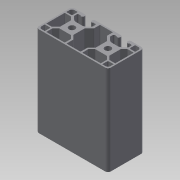
# Autodesk Inventor part: 40-4082-LITE
Saved by Autodesk Inventor 2013 (Build 170138000, 138)
## iProperties
Created: 2014-04-23
Part Number: 40-4082-LITE
Material: Generic
Document SubType Name: Modeling
Designer: Ross Bowman
Density: 1 g/cm^3
Engineer: Ross Bowman
Catalog Web Link: 8020.net
Vendor: 80/20 Inc.
Company: 80/20 Inc.
Author: Ross Bowman
Keywords: 80/20 , 8020 , T-Slot , Extrusion
Material: 6105-T5 Aluminum
Autodesk Inventor part; units mm, degrees
ref_plane "YZ Plane" through (0, 0, 0) normal (1, 0, 0) x (0, 1, 0)
ref_plane "XZ Plane" through (0, 0, 0) normal (0, 1, 0) x (-1, 0, 0)
ref_plane "XY Plane" through (0, 0, 0) normal (0, 0, 1) x (1, 0, 0)
sketch "Sketch1" plane through (0, 0, 0) normal (0, 0, 1) x (1, 0, 0)
  circle A0 centre (-20, 0) radius 3.3778
  circle A1 centre (20, 0) radius 3.3778
  arc A2 (31.462, -10.0253) -> (32.0906, -10.2857) centre (32.0906, -9.3967) ccw
  line L0 (27.9429, -6.5063) -> (31.462, -10.0253)
  arc A3 (27.6825, -5.8776) -> (27.9429, -6.5063) centre (28.5715, -5.8776) ccw
  line L1 (27.6825, 6.0573) -> (27.6825, -5.8776)
  arc A4 (27.9429, 6.6858) -> (27.6825, 6.0573) centre (28.5714, 6.0573) ccw
  line L2 (31.2824, 10.0254) -> (27.9429, 6.6858)
  arc A5 (31.911, 10.2857) -> (31.2824, 10.0254) centre (31.911, 9.3968) ccw
  line L3 (37.975, 10.2857) -> (31.911, 10.2857)
  line L4 (32.0906, -10.2857) -> (37.975, -10.2857)
  arc A6 (30.2857, -11.911) -> (30.0253, -11.2824) centre (29.3967, -11.911) ccw
  line L5 (30.2857, -17.975) -> (30.2857, -11.911)
  line L6 (9.7143, -11.911) -> (9.7143, -17.975)
  arc A7 (9.9746, -11.2824) -> (9.7143, -11.911) centre (10.6032, -11.911) ccw
  line L7 (13.3142, -7.9429) -> (9.9746, -11.2824)
  arc A8 (13.9427, -7.6825) -> (13.3142, -7.9429) centre (13.9427, -8.5714) ccw
  line L8 (26.0572, -7.6825) -> (13.9427, -7.6825)
  arc A9 (26.6858, -7.9429) -> (26.0572, -7.6825) centre (26.0572, -8.5715) ccw
  line L9 (30.0253, -11.2824) -> (26.6858, -7.9429)
  arc A10 (-26.0573, -7.6825) -> (-26.6858, -7.9429) centre (-26.0573, -8.5714) ccw
  line L10 (-13.9427, -7.6825) -> (-26.0573, -7.6825)
  arc A11 (-13.3142, -7.9429) -> (-13.9427, -7.6825) centre (-13.9427, -8.5714) ccw
  line L11 (-9.9746, -11.2824) -> (-13.3142, -7.9429)
  arc A12 (-9.7143, -11.911) -> (-9.9746, -11.2824) centre (-10.6032, -11.911) ccw
  line L12 (-9.7143, -17.975) -> (-9.7143, -11.911)
  line L13 (-30.2857, -11.911) -> (-30.2857, -17.975)
  arc A13 (-30.0254, -11.2824) -> (-30.2857, -11.911) centre (-29.3968, -11.911) ccw
  line L14 (-26.6858, -7.9429) -> (-30.0254, -11.2824)
  line L15 (-33.2063, -11.9365) -> (-37.975, -11.9365)
  arc A14 (-31.9365, -13.2063) -> (-33.2063, -11.9365) centre (-33.2063, -13.2063) ccw
  line L16 (-31.9365, -17.975) -> (-31.9365, -13.2063)
  line L17 (-31.9365, 13.2063) -> (-31.9365, 17.9355)
  arc A15 (-33.2063, 11.9365) -> (-31.9365, 13.2063) centre (-33.2063, 13.2063) ccw
  line L18 (-37.975, 11.9365) -> (-33.2063, 11.9365)
  arc A16 (-31.2824, 10.0254) -> (-31.911, 10.2857) centre (-31.911, 9.3968) ccw
  line L19 (-27.9429, 6.6858) -> (-31.2824, 10.0254)
  arc A17 (-27.6825, 6.0573) -> (-27.9429, 6.6858) centre (-28.5714, 6.0573) ccw
  line L20 (-27.6825, -5.5185) -> (-27.6825, 6.0573)
  arc A18 (-27.9429, -6.1471) -> (-27.6825, -5.5185) centre (-28.5714, -5.5185) ccw
  line L21 (-31.8212, -10.0254) -> (-27.9429, -6.1471)
  arc A19 (-32.4497, -10.2857) -> (-31.8212, -10.0254) centre (-32.4497, -9.3968) ccw
  line L22 (-37.975, -10.2857) -> (-32.4497, -10.2857)
  line L23 (-31.911, 10.2857) -> (-37.975, 10.2857)
  arc A20 (7.1746, 11.9365) -> (7.435, 11.308) centre (8.0635, 11.9365) ccw
  line L24 (12.0571, 6.6858) -> (7.435, 11.308)
  arc A21 (12.3175, 6.0573) -> (12.0571, 6.6858) centre (11.4286, 6.0573) ccw
  line L25 (12.3175, -5.8777) -> (12.3175, 6.0573)
  arc A22 (12.0571, -6.5062) -> (12.3175, -5.8777) centre (11.4286, -5.8777) ccw
  line L26 (8.0699, -10.4935) -> (12.0571, -6.5062)
  arc A23 (8.0699, -10.4935) -> (7.8095, -11.122) centre (8.6984, -11.122) ccw
  line L27 (7.8095, -17.975) -> (7.8095, -11.122)
  line L28 (-7.8095, -11.122) -> (-7.8095, -17.975)
  arc A24 (-7.8095, -11.122) -> (-8.0699, -10.4935) centre (-8.6984, -11.122) ccw
  line L29 (-12.0571, -6.5062) -> (-8.0699, -10.4935)
  arc A25 (-12.3175, -5.8777) -> (-12.0571, -6.5062) centre (-11.4286, -5.8777) ccw
  line L30 (-12.3175, 6.0573) -> (-12.3175, -5.8777)
  arc A26 (-12.0571, 6.6858) -> (-12.3175, 6.0573) centre (-11.4286, 6.0573) ccw
  line L31 (-7.435, 11.308) -> (-12.0571, 6.6858)
  arc A27 (-7.435, 11.308) -> (-7.1746, 11.9365) centre (-8.0635, 11.9365) ccw
  line L32 (-7.1746, 17.9355) -> (-7.1746, 11.9365)
  line L33 (35.56, 18.3105) -> (32.3115, 18.3105)
  line L34 (7.1746, 11.9365) -> (7.1746, 17.9355)
  line L35 (31.9365, -13.2063) -> (31.9365, -17.975)
  arc A28 (33.2063, -11.9365) -> (31.9365, -13.2063) centre (33.2063, -13.2063) ccw
  line L36 (37.975, -11.9365) -> (33.2063, -11.9365)
  line L37 (33.2063, 11.9365) -> (37.975, 11.9365)
  arc A29 (31.9365, 13.2063) -> (33.2063, 11.9365) centre (33.2063, 13.2063) ccw
  line L38 (31.9365, 17.9355) -> (31.9365, 13.2063)
  arc A30 (36.8254, -20) -> (40, -16.8254) centre (36.8254, -16.8254) ccw
  line L39 (40, -16.8254) -> (40, 16.8254)
  arc A31 (40, 16.8254) -> (36.8254, 20) centre (36.8254, 16.8254) ccw
  line L40 (36.8254, 20) -> (25.6381, 20)
  arc A32 (25.6381, 20) -> (24.0635, 18.4254) centre (25.6381, 18.4254) ccw
  line L41 (24.0635, 18.4254) -> (24.0635, 17.5111)
  arc A33 (24.0635, 17.5111) -> (25.6381, 15.9365) centre (25.6381, 17.5111) ccw
  line L42 (25.6381, 15.9365) -> (26.3446, 15.9365)
  arc A34 (26.3446, 15.9365) -> (26.7243, 16.3032) centre (26.3446, 16.3165) ccw
  line L43 (26.7243, 16.3032) -> (26.7253, 16.3317)
  arc A35 (27.105, 16.6984) -> (26.7253, 16.3317) centre (27.105, 16.3185) ccw
  line L44 (27.105, 16.6984) -> (29.0159, 16.6984)
  arc A36 (30.2857, 15.4286) -> (29.0159, 16.6984) centre (29.0159, 15.4286) ccw
  line L45 (30.2857, 15.4286) -> (30.2857, 12.9885)
  arc A37 (30.0254, 12.3599) -> (30.2857, 12.9885) centre (29.3968, 12.9885) ccw
  line L46 (30.0254, 12.3599) -> (26.739, 9.0736)
  arc A38 (23.3808, 7.6825) -> (26.739, 9.0736) centre (23.3808, 12.4317) ccw
  line L47 (23.3808, 7.6825) -> (16.6192, 7.6825)
  arc A39 (13.261, 9.0736) -> (16.6192, 7.6825) centre (16.6192, 12.4317) ccw
  line L48 (13.261, 9.0736) -> (9.9746, 12.3599)
  arc A40 (9.7143, 12.9885) -> (9.9746, 12.3599) centre (10.6032, 12.9885) ccw
  line L49 (9.7143, 12.9885) -> (9.7143, 15.4286)
  arc A41 (10.9841, 16.6984) -> (9.7143, 15.4286) centre (10.9841, 15.4286) ccw
  line L50 (10.9841, 16.6984) -> (12.895, 16.6984)
  arc A42 (13.2747, 16.3317) -> (12.895, 16.6984) centre (12.895, 16.3185) ccw
  line L51 (13.2747, 16.3317) -> (13.2757, 16.3032)
  arc A43 (13.2757, 16.3032) -> (13.6554, 15.9365) centre (13.6554, 16.3165) ccw
  line L52 (13.6554, 15.9365) -> (14.3619, 15.9365)
  arc A44 (14.3619, 15.9365) -> (15.9365, 17.5111) centre (14.3619, 17.5111) ccw
  line L53 (15.9365, 17.5111) -> (15.9365, 18.4254)
  arc A45 (15.9365, 18.4254) -> (14.3619, 20) centre (14.3619, 18.4254) ccw
  line L54 (14.3619, 20) -> (-14.3619, 20)
  arc A46 (-14.3619, 20) -> (-15.9365, 18.4254) centre (-14.3619, 18.4254) ccw
  line L55 (-15.9365, 18.4254) -> (-15.9365, 17.5111)
  arc A47 (-15.9365, 17.5111) -> (-14.3619, 15.9365) centre (-14.3619, 17.5111) ccw
  line L56 (-14.3619, 15.9365) -> (-13.6554, 15.9365)
  arc A48 (-13.6554, 15.9365) -> (-13.2757, 16.3032) centre (-13.6554, 16.3165) ccw
  line L57 (-13.2757, 16.3032) -> (-13.2747, 16.3317)
  arc A49 (-12.895, 16.6984) -> (-13.2747, 16.3317) centre (-12.895, 16.3185) ccw
  line L58 (-12.895, 16.6984) -> (-10.9841, 16.6984)
  arc A50 (-9.7143, 15.4286) -> (-10.9841, 16.6984) centre (-10.9841, 15.4286) ccw
  line L59 (-9.7143, 15.4286) -> (-9.7143, 12.9885)
  arc A51 (-9.9746, 12.3599) -> (-9.7143, 12.9885) centre (-10.6032, 12.9885) ccw
  line L60 (-9.9746, 12.3599) -> (-13.261, 9.0736)
  arc A52 (-16.6192, 7.6825) -> (-13.261, 9.0736) centre (-16.6192, 12.4317) ccw
  line L61 (-16.6192, 7.6825) -> (-23.3808, 7.6825)
  arc A53 (-26.739, 9.0736) -> (-23.3808, 7.6825) centre (-23.3808, 12.4317) ccw
  line L62 (-26.739, 9.0736) -> (-30.0254, 12.3599)
  arc A54 (-30.2857, 12.9885) -> (-30.0254, 12.3599) centre (-29.3968, 12.9885) ccw
  line L63 (-30.2857, 12.9885) -> (-30.2857, 15.4286)
  arc A55 (-29.0159, 16.6984) -> (-30.2857, 15.4286) centre (-29.0159, 15.4286) ccw
  line L64 (-29.0159, 16.6984) -> (-27.105, 16.6984)
  arc A56 (-26.7253, 16.3317) -> (-27.105, 16.6984) centre (-27.105, 16.3185) ccw
  line L65 (-26.7253, 16.3317) -> (-26.7243, 16.3032)
  arc A57 (-26.7243, 16.3032) -> (-26.3446, 15.9365) centre (-26.3446, 16.3165) ccw
  line L66 (-26.3446, 15.9365) -> (-25.6381, 15.9365)
  arc A58 (-25.6381, 15.9365) -> (-24.0635, 17.5111) centre (-25.6381, 17.5111) ccw
  line L67 (-24.0635, 17.5111) -> (-24.0635, 18.4254)
  arc A59 (-24.0635, 18.4254) -> (-25.6381, 20) centre (-25.6381, 18.4254) ccw
  line L68 (-25.6381, 20) -> (-36.8254, 20)
  arc A60 (-36.8254, 20) -> (-40, 16.8254) centre (-36.8254, 16.8254) ccw
  line L69 (-40, 16.8254) -> (-40, -16.8254)
  arc A61 (-40, -16.8254) -> (-36.8254, -20) centre (-36.8254, -16.8254) ccw
  line L70 (-36.8254, -20) -> (36.8254, -20)
  line L71 (-38.35, 15.5205) -> (-38.35, 12.3115)
  line L72 (-35.56, -18.35) -> (-32.3115, -18.35)
  line L73 (38.35, -15.56) -> (38.35, -12.3115)
  arc A62 (-38.35, -15.56) -> (-35.56, -18.35) centre (-35.56, -15.56) ccw
  arc A63 (-35.56, 18.3105) -> (-38.35, 15.5205) centre (-35.56, 15.5205) ccw
  arc A64 (38.35, 15.5205) -> (35.56, 18.3105) centre (35.56, 15.5205) ccw
  arc A65 (35.56, -18.35) -> (38.35, -15.56) centre (35.56, -15.56) ccw
  line L74 (-32.3115, 18.3105) -> (-35.56, 18.3105)
  line L75 (6.7996, 18.3105) -> (-6.7996, 18.3105)
  line L76 (38.35, 12.3115) -> (38.35, 15.5205)
  line L77 (38.35, -9.9107) -> (38.35, 9.9107)
  line L78 (32.3115, -18.35) -> (35.56, -18.35)
  line L79 (10.0893, -18.35) -> (29.9107, -18.35)
  line L80 (-7.4345, -18.35) -> (7.4345, -18.35)
  line L81 (-29.9107, -18.35) -> (-10.0893, -18.35)
  line L82 (-38.35, -12.3115) -> (-38.35, -15.56)
  line L83 (-38.35, 9.9107) -> (-38.35, -9.9107)
  arc A66 (-37.975, -11.9365) -> (-38.35, -12.3115) centre (-37.975, -12.3115) ccw
  arc A67 (-38.35, -9.9107) -> (-37.975, -10.2857) centre (-37.975, -9.9107) ccw
  arc A68 (-32.3115, -18.35) -> (-31.9365, -17.975) centre (-32.3115, -17.975) ccw
  arc A69 (-30.2857, -17.975) -> (-29.9107, -18.35) centre (-29.9107, -17.975) ccw
  arc A70 (-10.0893, -18.35) -> (-9.7143, -17.975) centre (-10.0893, -17.975) ccw
  arc A71 (-7.8095, -17.975) -> (-7.4345, -18.35) centre (-7.4345, -17.975) ccw
  arc A72 (7.4345, -18.35) -> (7.8095, -17.975) centre (7.4345, -17.975) ccw
  arc A73 (9.7143, -17.975) -> (10.0893, -18.35) centre (10.0893, -17.975) ccw
  arc A74 (29.9107, -18.35) -> (30.2857, -17.975) centre (29.9107, -17.975) ccw
  arc A75 (31.9365, -17.975) -> (32.3115, -18.35) centre (32.3115, -17.975) ccw
  arc A76 (38.35, -12.3115) -> (37.975, -11.9365) centre (37.975, -12.3115) ccw
  arc A77 (37.975, -10.2857) -> (38.35, -9.9107) centre (37.975, -9.9107) ccw
  arc A78 (38.35, 9.9107) -> (37.975, 10.2857) centre (37.975, 9.9107) ccw
  arc A79 (37.975, 11.9365) -> (38.35, 12.3115) centre (37.975, 12.3115) ccw
  arc A80 (32.3115, 18.3105) -> (31.9365, 17.9355) centre (32.3115, 17.9355) ccw
  arc A81 (7.1746, 17.9355) -> (6.7996, 18.3105) centre (6.7996, 17.9355) ccw
  arc A82 (-6.7996, 18.3105) -> (-7.1746, 17.9355) centre (-6.7996, 17.9355) ccw
  arc A83 (-31.9365, 17.9355) -> (-32.3115, 18.3105) centre (-32.3115, 17.9355) ccw
  arc A84 (-38.35, 12.3115) -> (-37.975, 11.9365) centre (-37.975, 12.3115) ccw
  arc A85 (-37.975, 10.2857) -> (-38.35, 9.9107) centre (-37.975, 9.9107) ccw
  point P0 (0, 0)
  constraints: 168 end point, 168 point on circle, 86 centre point
extrude "Extrusion1" add sketch "Sketch1" against normal blind 100
body "Solid1"
